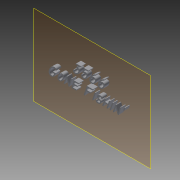
# Autodesk Inventor part: RaisedLetters3566GF
Saved by Autodesk Inventor 2015 (Build 190159000, 159)
## iProperties
Created: 2016-02-29
Part Number: RaisedLetters3566GF
Material: Generic
Document SubType Name: Modeling
Designer: robotics
Density: 1 g/cm^3
Appearance: Default
Author: robotics
Autodesk Inventor part; units mm, degrees
ref_plane "YZ Plane" through (0, 0, 0) normal (1, 0, 0) x (0, 1, 0)
ref_plane "XZ Plane" through (0, 0, 0) normal (0, 1, 0) x (-1, 0, 0)
ref_plane "XY Plane" through (0, 0, 0) normal (0, 0, 1) x (1, 0, 0)
sketch "Sketch1" plane through (0, 0, 0) normal (0, 0, 1) x (1, 0, 0)
  line L0 (0, 0) -> (127, 0)
  line L1 (127, 0) -> (127, 76.2)
  line L2 (127, 76.2) -> (0, 76.2)
  line L3 (0, 76.2) -> (0, 0)
  line L4 (3.7507, 56.7748) -> (124.5302, 56.7748) construction
  line L5 (124.5302, 56.7748) -> (124.5302, -11.4457) construction
  line L6 (124.5302, -11.4457) -> (3.7507, -11.4457) construction
  line L7 (3.7507, -11.4457) -> (3.7507, 56.7748) construction
  spline S0 degree 2 poles (52.7475, 48.5617) (52.0257, 46.4353) (50.3285, 45.138) knots 0 0 0 1 1 1
  spline S1 degree 2 poles (50.3285, 45.138) (48.7873, 43.9772) (47.1681, 43.9772) knots 0 0 0 1 1 1
  spline S2 degree 2 poles (47.1681, 43.9772) (45.9098, 43.9772) (45.1685, 44.7186) knots 0 0 0 1 1 1
  spline S3 degree 2 poles (45.1685, 44.7186) (44.3491, 45.5282) (44.3882, 46.9913) knots 0 0 0 1 1 1
  spline S4 degree 2 poles (44.3882, 46.9913) (44.3979, 47.1181) (44.4369, 47.2449) knots 0 0 0 1 1 1
  spline S5 degree 2 poles (44.4369, 47.2449) (44.554, 47.5765) (45.149, 47.9862) (45.4416, 47.9862) knots 0 0 0 1 2 2 2
  spline S6 degree 2 poles (45.4416, 47.9862) (45.9586, 47.9862) (45.9488, 47.4692) knots 0 0 0 1 1 1
  spline S7 degree 2 poles (45.9488, 47.4692) (45.9196, 46.5621) (46.4268, 46.0451) knots 0 0 0 1 1 1
  spline S8 degree 2 poles (46.4268, 46.0451) (46.9048, 45.5867) (47.6753, 45.5867) knots 0 0 0 1 1 1
  spline S9 degree 2 poles (47.6753, 45.5867) (48.7093, 45.5867) (49.714, 46.3573) knots 0 0 0 1 1 1
  spline S10 degree 2 poles (49.714, 46.3573) (50.8064, 47.1961) (51.2746, 48.5617) knots 0 0 0 1 1 1
  spline S11 degree 2 poles (51.2746, 48.5617) (51.7721, 50.0151) (51.1771, 50.7759) knots 0 0 0 1 1 1
  spline S12 degree 2 poles (51.1771, 50.7759) (50.7284, 51.3027) (49.7335, 51.4685) knots 0 0 0 1 1 1
  spline S13 degree 2 poles (49.7335, 51.4685) (49.1872, 51.5075) (48.6313, 51.5465) knots 0 0 0 1 1 1
  spline S14 degree 2 poles (48.6313, 51.5465) (48.3289, 51.566) (48.046, 51.9562) (48.1143, 52.1513) knots 0 0 0 1 2 2 2
  spline S15 degree 2 poles (48.1143, 52.1513) (48.2411, 52.5219) (48.6703, 52.8536) knots 0 0 0 1 1 1
  line L8 (48.6703, 52.8536) -> (51.577, 55.1068)
  line L9 (51.577, 55.1068) -> (48.3874, 55.1068)
  spline S16 degree 2 poles (48.3874, 55.1068) (47.6461, 55.1068) (47.8997, 55.8676) knots 0 0 0 1 1 1
  spline S17 degree 2 poles (47.8997, 55.8676) (48.163, 56.6382) (48.9044, 56.6382) knots 0 0 0 1 1 1
  line L10 (48.9044, 56.6382) -> (54.5033, 56.6577)
  spline S18 degree 2 poles (54.5033, 56.6577) (55.0203, 56.6577) (54.8935, 56.2773) knots 0 0 0 1 1 1
  spline S19 degree 2 poles (54.8935, 56.2773) (54.7959, 55.9944) (53.8888, 55.3019) knots 0 0 0 1 1 1
  line L11 (53.8888, 55.3019) -> (50.904, 52.9706)
  spline S20 degree 2 poles (50.904, 52.9706) (54.0156, 52.3073) (52.7475, 48.5617) knots 0 0 0 1 1 1
  spline S21 degree 2 poles (63.1065, 48.4056) (62.4725, 46.5426) (61.2044, 45.3623) knots 0 0 0 1 1 1
  spline S22 degree 2 poles (61.2044, 45.3623) (59.8096, 44.0845) (57.9758, 43.9577) knots 0 0 0 1 1 1
  spline S23 degree 2 poles (57.9758, 43.9577) (56.5322, 43.8504) (55.7421, 44.7673) knots 0 0 0 1 1 1
  spline S24 degree 2 poles (55.7421, 44.7673) (55.0105, 45.6062) (55.0008, 47.0401) knots 0 0 0 1 1 1
  spline S25 degree 2 poles (55.0008, 47.0401) (54.991, 47.1864) (55.0398, 47.3327) knots 0 0 0 1 1 1
  spline S26 degree 2 poles (55.0398, 47.3327) (55.1471, 47.6546) (55.7713, 48.074) (56.0835, 48.074) knots 0 0 0 1 2 2 2
  spline S27 degree 2 poles (56.0835, 48.074) (56.5712, 48.074) (56.5809, 47.5765) knots 0 0 0 1 1 1
  spline S28 degree 2 poles (56.5809, 47.5765) (56.6395, 45.4013) (58.4147, 45.5086) knots 0 0 0 1 1 1
  spline S29 degree 2 poles (58.4147, 45.5086) (59.5462, 45.5867) (60.4241, 46.4353) knots 0 0 0 1 1 1
  spline S30 degree 2 poles (60.4241, 46.4353) (61.224, 47.2059) (61.6336, 48.4056) knots 0 0 0 1 1 1
  spline S31 degree 2 poles (61.6336, 48.4056) (62.0238, 49.5762) (61.1264, 51.2734) (60.151, 51.2734) knots 0 0 0 1 2 2 2
  spline S32 degree 2 poles (60.151, 51.2734) (58.8049, 51.2734) (57.7222, 50.5906) knots 0 0 0 1 1 1
  spline S33 degree 2 poles (57.7222, 50.5906) (57.176, 50.2394) (56.9028, 50.2394) knots 0 0 0 1 1 1
  spline S34 degree 2 poles (56.9028, 50.2394) (56.2883, 50.2394) (56.5224, 50.9222) knots 0 0 0 1 1 1
  line L12 (56.5224, 50.9222) -> (58.4733, 56.648)
  line L13 (58.4733, 56.648) -> (64.2283, 56.648)
  spline S35 degree 2 poles (64.2283, 56.648) (64.9793, 56.648) (64.7257, 55.8871) knots 0 0 0 1 1 1
  spline S36 degree 2 poles (64.7257, 55.8871) (64.4624, 55.1166) (63.7015, 55.1166) knots 0 0 0 1 1 1
  line L14 (63.7015, 55.1166) -> (59.4194, 55.1166)
  line L15 (59.4194, 55.1166) -> (58.522, 52.4537)
  spline S37 degree 2 poles (58.522, 52.4537) (59.4877, 52.8243) (60.6777, 52.8243) knots 0 0 0 1 1 1
  spline S38 degree 2 poles (60.6777, 52.8243) (62.2091, 52.8243) (63.7113, 50.2004) (63.1065, 48.4056) knots 0 0 0 1 2 2 2
  spline S39 degree 2 poles (74.4604, 48.5715) (73.7679, 46.5231) (70.6758, 43.8992) (68.9103, 43.8992) knots 0 0 0 1 2 2 2
  spline S40 degree 2 poles (68.9103, 43.8992) (66.6961, 43.8992) (66.0425, 45.4696) knots 0 0 0 1 1 1
  spline S41 degree 2 poles (66.0425, 45.4696) (65.4573, 46.8352) (66.1889, 49.0007) knots 0 0 0 1 1 1
  spline S42 degree 2 poles (66.1889, 49.0007) (66.5693, 50.1224) (67.2618, 51.2344) knots 0 0 0 1 1 1
  spline S43 degree 2 poles (67.2618, 51.2344) (68.3543, 52.9706) (69.7101, 54.1899) knots 0 0 0 1 1 1
  spline S44 degree 2 poles (69.7101, 54.1899) (71.1928, 55.5165) (73.485, 56.6675) knots 0 0 0 1 1 1
  spline S45 degree 2 poles (73.485, 56.6675) (73.7094, 56.7748) (73.8947, 56.7748) knots 0 0 0 1 1 1
  spline S46 degree 2 poles (73.8947, 56.7748) (74.2068, 56.7748) (74.4604, 56.2773) (74.3531, 55.9652) knots 0 0 0 1 2 2 2
  spline S47 degree 2 poles (74.3531, 55.9652) (74.2068, 55.536) (73.7679, 55.3116) knots 0 0 0 1 1 1
  spline S48 degree 2 poles (73.7679, 55.3116) (72.4511, 54.6484) (71.4952, 53.907) knots 0 0 0 1 1 1
  spline S49 degree 2 poles (71.4952, 53.907) (70.6563, 53.2828) (69.515, 52.1415) knots 0 0 0 1 1 1
  spline S50 degree 2 poles (69.515, 52.1415) (70.5783, 52.6878) (71.7975, 52.6878) knots 0 0 0 1 1 1
  spline S51 degree 2 poles (71.7975, 52.6878) (73.7191, 52.6878) (75.1237, 50.5321) (74.4604, 48.5715) knots 0 0 0 1 2 2 2
  spline S52 degree 2 poles (72.968, 48.5715) (73.3289, 49.6249) (72.3243, 51.1368) (71.2708, 51.1368) knots 0 0 0 1 2 2 2
  spline S53 degree 2 poles (71.2708, 51.1368) (70.1491, 51.1368) (67.9934, 49.4786) (67.5935, 48.2984) knots 0 0 0 1 2 2 2
  spline S54 degree 2 poles (67.5935, 48.2984) (67.1838, 47.1083) (68.2665, 45.4501) (69.437, 45.4501) knots 0 0 0 1 2 2 2
  spline S55 degree 2 poles (69.437, 45.4501) (70.5197, 45.4501) (71.5732, 46.4255) knots 0 0 0 1 1 1
  spline S56 degree 2 poles (71.5732, 46.4255) (72.5486, 47.3327) (72.968, 48.5715) knots 0 0 0 1 1 1
  spline S57 degree 2 poles (85.5705, 48.5715) (84.8779, 46.5231) (81.7859, 43.8992) (80.0203, 43.8992) knots 0 0 0 1 2 2 2
  spline S58 degree 2 poles (80.0203, 43.8992) (77.8061, 43.8992) (77.1526, 45.4696) knots 0 0 0 1 1 1
  spline S59 degree 2 poles (77.1526, 45.4696) (76.5673, 46.8352) (77.2989, 49.0007) knots 0 0 0 1 1 1
  spline S60 degree 2 poles (77.2989, 49.0007) (77.6793, 50.1224) (78.3719, 51.2344) knots 0 0 0 1 1 1
  spline S61 degree 2 poles (78.3719, 51.2344) (79.4644, 52.9706) (80.8202, 54.1899) knots 0 0 0 1 1 1
  spline S62 degree 2 poles (80.8202, 54.1899) (82.3028, 55.5165) (84.5951, 56.6675) knots 0 0 0 1 1 1
  spline S63 degree 2 poles (84.5951, 56.6675) (84.8194, 56.7748) (85.0048, 56.7748) knots 0 0 0 1 1 1
  spline S64 degree 2 poles (85.0048, 56.7748) (85.3169, 56.7748) (85.5705, 56.2773) (85.4632, 55.9652) knots 0 0 0 1 2 2 2
  spline S65 degree 2 poles (85.4632, 55.9652) (85.3169, 55.536) (84.8779, 55.3116) knots 0 0 0 1 1 1
  spline S66 degree 2 poles (84.8779, 55.3116) (83.5611, 54.6484) (82.6052, 53.907) knots 0 0 0 1 1 1
  spline S67 degree 2 poles (82.6052, 53.907) (81.7664, 53.2828) (80.6251, 52.1415) knots 0 0 0 1 1 1
  spline S68 degree 2 poles (80.6251, 52.1415) (81.6883, 52.6878) (82.9076, 52.6878) knots 0 0 0 1 1 1
  spline S69 degree 2 poles (82.9076, 52.6878) (84.8292, 52.6878) (86.2338, 50.5321) (85.5705, 48.5715) knots 0 0 0 1 2 2 2
  spline S70 degree 2 poles (84.0781, 48.5715) (84.439, 49.6249) (83.4343, 51.1368) (82.3809, 51.1368) knots 0 0 0 1 2 2 2
  spline S71 degree 2 poles (82.3809, 51.1368) (81.2591, 51.1368) (79.1034, 49.4786) (78.7035, 48.2984) knots 0 0 0 1 2 2 2
  spline S72 degree 2 poles (78.7035, 48.2984) (78.2938, 47.1083) (79.3766, 45.4501) (80.5471, 45.4501) knots 0 0 0 1 2 2 2
  spline S73 degree 2 poles (80.5471, 45.4501) (81.6298, 45.4501) (82.6832, 46.4255) knots 0 0 0 1 1 1
  spline S74 degree 2 poles (82.6832, 46.4255) (83.6587, 47.3327) (84.0781, 48.5715) knots 0 0 0 1 1 1
  spline S75 degree 2 poles (20.9439, 30.1166) (20.0758, 27.5708) (18.2712, 26.332) knots 0 0 0 1 1 1
  spline S76 degree 2 poles (18.2712, 26.332) (16.9934, 25.4638) (15.7059, 25.4638) knots 0 0 0 1 1 1
  spline S77 degree 2 poles (15.7059, 25.4638) (13.4819, 25.4638) (12.7211, 27.5122) knots 0 0 0 1 1 1
  spline S78 degree 2 poles (12.7211, 27.5122) (12.009, 29.3753) (12.8284, 31.8041) knots 0 0 0 1 1 1
  spline S79 degree 2 poles (12.8284, 31.8041) (13.8428, 34.7694) (15.8619, 36.5837) knots 0 0 0 1 1 1
  spline S80 degree 2 poles (15.8619, 36.5837) (17.7835, 38.3394) (19.8709, 38.3394) knots 0 0 0 1 1 1
  spline S81 degree 2 poles (19.8709, 38.3394) (21.3341, 38.3394) (22.0071, 37.7347) knots 0 0 0 1 1 1
  spline S82 degree 2 poles (22.0071, 37.7347) (22.407, 37.3835) (22.6996, 36.4569) knots 0 0 0 1 1 1
  spline S83 degree 2 poles (22.6996, 36.4569) (22.7874, 36.213) (22.6996, 35.9594) knots 0 0 0 1 1 1
  spline S84 degree 2 poles (22.6996, 35.9594) (22.6021, 35.657) (21.9973, 35.2376) (21.695, 35.2376) knots 0 0 0 1 2 2 2
  spline S85 degree 2 poles (21.695, 35.2376) (21.3145, 35.2376) (21.1682, 35.5887) knots 0 0 0 1 1 1
  spline S86 degree 2 poles (21.1682, 35.5887) (20.9244, 36.2325) (20.6805, 36.4373) knots 0 0 0 1 1 1
  spline S87 degree 2 poles (20.6805, 36.4373) (20.2904, 36.7885) (19.3442, 36.7885) knots 0 0 0 1 1 1
  spline S88 degree 2 poles (19.3442, 36.7885) (17.8518, 36.7885) (15.1011, 34.0378) (14.3403, 31.8041) knots 0 0 0 1 2 2 2
  spline S89 degree 2 poles (14.3403, 31.8041) (13.7258, 29.9898) (14.1549, 28.5852) knots 0 0 0 1 1 1
  spline S90 degree 2 poles (14.1549, 28.5852) (14.6427, 27.0148) (16.2228, 27.0148) knots 0 0 0 1 1 1
  spline S91 degree 2 poles (16.2228, 27.0148) (17.6274, 27.0148) (18.5346, 28.3804) knots 0 0 0 1 1 1
  spline S92 degree 2 poles (18.5346, 28.3804) (19.0223, 29.0827) (19.5198, 30.5653) knots 0 0 0 1 1 1
  line L16 (19.5198, 30.5653) -> (17.842, 30.5653)
  spline S93 degree 2 poles (17.842, 30.5653) (17.0617, 30.5653) (17.3251, 31.3456) knots 0 0 0 1 1 1
  spline S94 degree 2 poles (17.3251, 31.3456) (17.5884, 32.1162) (18.3688, 32.1162) knots 0 0 0 1 1 1
  line L17 (18.3688, 32.1162) -> (21.6169, 32.1162)
  line L18 (21.6169, 32.1162) -> (20.9439, 30.1166)
  spline S95 degree 2 poles (32.0344, 30.7506) (31.3419, 28.7218) (29.8007, 27.1806) knots 0 0 0 1 1 1
  spline S96 degree 2 poles (29.8007, 27.1806) (28.1327, 25.5224) (26.416, 25.5224) knots 0 0 0 1 1 1
  spline S97 degree 2 poles (26.416, 25.5224) (24.6993, 25.5224) (24.1628, 27.2001) knots 0 0 0 1 1 1
  spline S98 degree 2 poles (24.1628, 27.2001) (23.6751, 28.7315) (24.3579, 30.7506) knots 0 0 0 1 1 1
  spline S99 degree 2 poles (24.3579, 30.7506) (25.0407, 32.76) (26.6013, 34.2719) knots 0 0 0 1 1 1
  spline S100 degree 2 poles (26.6013, 34.2719) (28.2888, 35.9204) (29.947, 35.9204) knots 0 0 0 1 1 1
  spline S101 degree 2 poles (29.947, 35.9204) (31.7223, 35.9204) (32.249, 34.2719) knots 0 0 0 1 1 1
  spline S102 degree 2 poles (32.249, 34.2719) (32.727, 32.799) (32.0344, 30.7506) knots 0 0 0 1 1 1
  spline S103 degree 2 poles (30.5615, 30.7506) (31.059, 32.2138) (30.8542, 33.2087) knots 0 0 0 1 1 1
  spline S104 degree 2 poles (30.8542, 33.2087) (30.6201, 34.4085) (29.4398, 34.4085) knots 0 0 0 1 1 1
  spline S105 degree 2 poles (29.4398, 34.4085) (28.3083, 34.4085) (27.2354, 33.2087) knots 0 0 0 1 1 1
  spline S106 degree 2 poles (27.2354, 33.2087) (26.3087, 32.1748) (25.8308, 30.7506) knots 0 0 0 1 1 1
  spline S107 degree 2 poles (25.8308, 30.7506) (25.343, 29.3265) (25.5576, 28.2731) knots 0 0 0 1 1 1
  spline S108 degree 2 poles (25.5576, 28.2731) (25.7917, 27.0538) (26.933, 27.0538) knots 0 0 0 1 1 1
  spline S109 degree 2 poles (26.933, 27.0538) (28.084, 27.0538) (29.1472, 28.2731) knots 0 0 0 1 1 1
  spline S110 degree 2 poles (29.1472, 28.2731) (30.0738, 29.3265) (30.5615, 30.7506) knots 0 0 0 1 1 1
  spline S111 degree 2 poles (39.8086, 26.3515) (39.5354, 25.5614) (38.9112, 25.5614) knots 0 0 0 1 1 1
  spline S112 degree 2 poles (38.9112, 25.5614) (38.4625, 25.5614) (38.2869, 26.0784) knots 0 0 0 1 1 1
  line L19 (38.2869, 26.0784) -> (35.9654, 32.8966)
  line L20 (35.9654, 32.8966) -> (33.7414, 26.332)
  spline S113 degree 2 poles (33.7414, 26.332) (33.4781, 25.5614) (32.7367, 25.5614) knots 0 0 0 1 1 1
  spline S114 degree 2 poles (32.7367, 25.5614) (32.0052, 25.5614) (32.2685, 26.332) knots 0 0 0 1 1 1
  line L21 (32.2685, 26.332) -> (35.2923, 35.2376)
  spline S115 degree 2 poles (35.2923, 35.2376) (35.546, 35.9887) (36.2483, 35.9887) knots 0 0 0 1 1 1
  spline S116 degree 2 poles (36.2483, 35.9887) (36.697, 35.9887) (36.853, 35.5302) knots 0 0 0 1 1 1
  line L22 (36.853, 35.5302) -> (39.155, 28.7705)
  line L23 (39.155, 28.7705) -> (41.3205, 35.1595)
  spline S117 degree 2 poles (41.3205, 35.1595) (41.5936, 35.9399) (42.3251, 35.9399) knots 0 0 0 1 1 1
  spline S118 degree 2 poles (42.3251, 35.9399) (43.0665, 35.9399) (42.7933, 35.1595) knots 0 0 0 1 1 1
  line L24 (42.7933, 35.1595) -> (39.8086, 26.3515)
  line L25 (48.0801, 25.7077) -> (42.0423, 25.7077)
  line L26 (42.0423, 25.7077) -> (45.5245, 35.9399)
  line L27 (45.5245, 35.9399) -> (51.5624, 35.9399)
  spline S119 degree 2 poles (51.5624, 35.9399) (52.3135, 35.9399) (52.0599, 35.1888) knots 0 0 0 1 1 1
  spline S120 degree 2 poles (52.0599, 35.1888) (51.7965, 34.428) (51.0454, 34.428) knots 0 0 0 1 1 1
  line L28 (51.0454, 34.428) -> (46.4707, 34.428)
  line L29 (46.4707, 34.428) -> (45.6806, 32.1162)
  line L30 (45.6806, 32.1162) -> (49.9822, 32.1162)
  spline S121 degree 2 poles (49.9822, 32.1162) (50.7235, 32.1162) (50.4602, 31.3554) knots 0 0 0 1 1 1
  spline S122 degree 2 poles (50.4602, 31.3554) (50.1968, 30.5848) (49.4652, 30.5848) knots 0 0 0 1 1 1
  line L31 (49.4652, 30.5848) -> (45.1636, 30.5848)
  line L32 (45.1636, 30.5848) -> (44.0224, 27.2391)
  line L33 (44.0224, 27.2391) -> (48.5971, 27.2391)
  spline S123 degree 2 poles (48.5971, 27.2391) (49.3579, 27.2391) (49.1043, 26.4783) knots 0 0 0 1 1 1
  spline S124 degree 2 poles (49.1043, 26.4783) (48.841, 25.7077) (48.0801, 25.7077) knots 0 0 0 1 1 1
  line L34 (69.5687, 36.6617) -> (63.5113, 36.6617)
  line L35 (63.5113, 36.6617) -> (62.3798, 33.355)
  line L36 (62.3798, 33.355) -> (67.0228, 33.355)
  spline S125 degree 2 poles (67.0228, 33.355) (67.7837, 33.355) (67.5203, 32.5844) knots 0 0 0 1 1 1
  spline S126 degree 2 poles (67.5203, 32.5844) (67.2472, 31.8041) (66.4961, 31.8041) knots 0 0 0 1 1 1
  line L37 (66.4961, 31.8041) -> (61.8531, 31.8041)
  line L38 (61.8531, 31.8041) -> (60.0193, 26.3905)
  spline S127 degree 2 poles (60.0193, 26.3905) (59.7462, 25.6004) (59.0146, 25.6004) knots 0 0 0 1 1 1
  spline S128 degree 2 poles (59.0146, 25.6004) (58.2538, 25.6004) (58.5269, 26.3905) knots 0 0 0 1 1 1
  line L39 (58.5269, 26.3905) -> (62.5457, 38.2126)
  line L40 (62.5457, 38.2126) -> (70.0954, 38.2126)
  spline S129 degree 2 poles (70.0954, 38.2126) (70.8562, 38.2126) (70.5929, 37.442) knots 0 0 0 1 1 1
  spline S130 degree 2 poles (70.5929, 37.442) (70.3198, 36.6617) (69.5687, 36.6617) knots 0 0 0 1 1 1
  spline S131 degree 2 poles (71.0904, 26.3612) (70.827, 25.5809) (70.0662, 25.5809) knots 0 0 0 1 1 1
  spline S132 degree 2 poles (70.0662, 25.5809) (69.3151, 25.5809) (69.5784, 26.3612) knots 0 0 0 1 1 1
  line L41 (69.5784, 26.3612) -> (72.573, 35.1791)
  spline S133 degree 2 poles (72.573, 35.1791) (72.8364, 35.9594) (73.5972, 35.9594) knots 0 0 0 1 1 1
  spline S134 degree 2 poles (73.5972, 35.9594) (74.3483, 35.9594) (74.0849, 35.1791) knots 0 0 0 1 1 1
  line L42 (74.0849, 35.1791) -> (71.0904, 26.3612)
  spline S135 degree 2 poles (81.4103, 28.5169) (80.3861, 25.5029) (76.6503, 25.5029) knots 0 0 0 1 1 1
  spline S136 degree 2 poles (76.6503, 25.5029) (74.5433, 25.5029) (74.1044, 27.7171) knots 0 0 0 1 1 1
  spline S137 degree 2 poles (74.1044, 27.7171) (74.0654, 27.8829) (74.1239, 28.0682) knots 0 0 0 1 1 1
  spline S138 degree 2 poles (74.1239, 28.0682) (74.2507, 28.4194) (74.9628, 28.9559) (75.2749, 28.9559) knots 0 0 0 1 2 2 2
  spline S139 degree 2 poles (75.2749, 28.9559) (75.6261, 28.9559) (75.6651, 28.5657) knots 0 0 0 1 1 1
  spline S140 degree 2 poles (75.6651, 28.5657) (75.7724, 27.0343) (77.177, 27.0343) knots 0 0 0 1 1 1
  spline S141 degree 2 poles (77.177, 27.0343) (79.3912, 27.0343) (79.8887, 28.4974) knots 0 0 0 1 1 1
  spline S142 degree 2 poles (79.8887, 28.4974) (80.113, 29.1607) (78.9035, 29.7655) knots 0 0 0 1 1 1
  spline S143 degree 2 poles (78.9035, 29.7655) (76.9819, 30.7116) (76.66, 30.975) knots 0 0 0 1 1 1
  spline S144 degree 2 poles (76.66, 30.975) (75.5578, 31.8919) (76.0553, 33.3745) knots 0 0 0 1 1 1
  spline S145 degree 2 poles (76.0553, 33.3745) (76.9429, 35.9984) (80.152, 36.1447) knots 0 0 0 1 1 1
  spline S146 degree 2 poles (80.152, 36.1447) (81.3713, 36.2032) (82.8735, 35.0522) (82.8539, 33.9305) knots 0 0 0 1 2 2 2
  spline S147 degree 2 poles (82.8539, 33.9305) (82.8539, 33.794) (82.8052, 33.6671) knots 0 0 0 1 1 1
  spline S148 degree 2 poles (82.8052, 33.6671) (82.7076, 33.3745) (82.1321, 32.9844) (81.8298, 32.9844) knots 0 0 0 1 2 2 2
  spline S149 degree 2 poles (81.8298, 32.9844) (81.2933, 32.9844) (81.3128, 34.0573) (80.4154, 34.6718) (79.7131, 34.6328) knots 0 0 0 1 2 3 3 3
  spline S150 degree 2 poles (79.7131, 34.6328) (77.9671, 34.5548) (77.5769, 33.4135) knots 0 0 0 1 1 1
  spline S151 degree 2 poles (77.5769, 33.4135) (77.2648, 32.4869) (78.4743, 31.8626) knots 0 0 0 1 1 1
  spline S152 degree 2 poles (78.4743, 31.8626) (79.6058, 31.3066) (80.7373, 30.7311) knots 0 0 0 1 1 1
  spline S153 degree 2 poles (80.7373, 30.7311) (81.8883, 29.9215) (81.4103, 28.5169) knots 0 0 0 1 1 1
  spline S154 degree 2 poles (89.994, 26.3612) (89.7307, 25.5809) (88.9894, 25.5809) knots 0 0 0 1 1 1
  spline S155 degree 2 poles (88.9894, 25.5809) (88.2383, 25.5809) (88.5016, 26.3515) knots 0 0 0 1 1 1
  line L43 (88.5016, 26.3515) -> (89.838, 30.3019)
  line L44 (89.838, 30.3019) -> (85.7314, 30.3019)
  line L45 (85.7314, 30.3019) -> (84.3951, 26.3515)
  spline S156 degree 2 poles (84.3951, 26.3515) (84.1317, 25.5809) (83.3709, 25.5809) knots 0 0 0 1 1 1
  spline S157 degree 2 poles (83.3709, 25.5809) (82.6198, 25.5809) (82.8832, 26.3612) knots 0 0 0 1 1 1
  line L46 (82.8832, 26.3612) -> (85.8778, 35.1791)
  spline S158 degree 2 poles (85.8778, 35.1791) (86.1411, 35.9594) (86.9019, 35.9594) knots 0 0 0 1 1 1
  spline S159 degree 2 poles (86.9019, 35.9594) (87.653, 35.9594) (87.3897, 35.1791) knots 0 0 0 1 1 1
  line L47 (87.3897, 35.1791) -> (86.2484, 31.8334)
  line L48 (86.2484, 31.8334) -> (90.3549, 31.8334)
  line L49 (90.3549, 31.8334) -> (91.4962, 35.1791)
  spline S160 degree 2 poles (91.4962, 35.1791) (91.7596, 35.9594) (92.5204, 35.9594) knots 0 0 0 1 1 1
  spline S161 degree 2 poles (92.5204, 35.9594) (93.2519, 35.9594) (92.9886, 35.1791) knots 0 0 0 1 1 1
  line L50 (92.9886, 35.1791) -> (89.994, 26.3612)
  spline S162 degree 2 poles (94.0908, 26.3612) (93.8274, 25.5809) (93.0666, 25.5809) knots 0 0 0 1 1 1
  spline S163 degree 2 poles (93.0666, 25.5809) (92.3155, 25.5809) (92.5789, 26.3612) knots 0 0 0 1 1 1
  line L51 (92.5789, 26.3612) -> (95.5735, 35.1791)
  spline S164 degree 2 poles (95.5735, 35.1791) (95.8368, 35.9594) (96.5976, 35.9594) knots 0 0 0 1 1 1
  spline S165 degree 2 poles (96.5976, 35.9594) (97.3487, 35.9594) (97.0854, 35.1791) knots 0 0 0 1 1 1
  line L52 (97.0854, 35.1791) -> (94.0908, 26.3612)
  spline S166 degree 2 poles (104.3327, 26.3515) (104.0596, 25.5614) (103.4354, 25.5614) knots 0 0 0 1 1 1
  spline S167 degree 2 poles (103.4354, 25.5614) (102.9867, 25.5614) (102.8111, 26.0784) knots 0 0 0 1 1 1
  line L53 (102.8111, 26.0784) -> (100.4896, 32.8966)
  line L54 (100.4896, 32.8966) -> (98.2656, 26.332)
  spline S168 degree 2 poles (98.2656, 26.332) (98.0023, 25.5614) (97.2609, 25.5614) knots 0 0 0 1 1 1
  spline S169 degree 2 poles (97.2609, 25.5614) (96.5294, 25.5614) (96.7927, 26.332) knots 0 0 0 1 1 1
  line L55 (96.7927, 26.332) -> (99.8165, 35.2376)
  spline S170 degree 2 poles (99.8165, 35.2376) (100.0702, 35.9887) (100.7725, 35.9887) knots 0 0 0 1 1 1
  spline S171 degree 2 poles (100.7725, 35.9887) (101.2211, 35.9887) (101.3772, 35.5302) knots 0 0 0 1 1 1
  line L56 (101.3772, 35.5302) -> (103.6792, 28.7705)
  line L57 (103.6792, 28.7705) -> (105.8447, 35.1595)
  spline S172 degree 2 poles (105.8447, 35.1595) (106.1178, 35.9399) (106.8493, 35.9399) knots 0 0 0 1 1 1
  spline S173 degree 2 poles (106.8493, 35.9399) (107.5907, 35.9399) (107.3175, 35.1595) knots 0 0 0 1 1 1
  line L58 (107.3175, 35.1595) -> (104.3327, 26.3515)
  spline S174 degree 2 poles (111.8337, 34.7401) (111.5996, 34.0573) (110.8388, 34.0573) knots 0 0 0 1 1 1
  spline S175 degree 2 poles (110.8388, 34.0573) (110.0877, 34.0573) (110.3218, 34.7401) knots 0 0 0 1 1 1
  line L59 (110.3218, 34.7401) -> (111.268, 37.5396)
  spline S176 degree 2 poles (111.268, 37.5396) (111.5021, 38.2224) (112.2629, 38.2224) knots 0 0 0 1 1 1
  spline S177 degree 2 poles (112.2629, 38.2224) (113.014, 38.2224) (112.7799, 37.5396) knots 0 0 0 1 1 1
  line L60 (112.7799, 37.5396) -> (111.8337, 34.7401)
  dimension "d0" = 127
  dimension "d1" = 76.2
  constraints: 8 end point, 2 parallel, 1 horizontal, 1 perpendicular, 2 other
  measures "d0" distance of L1.end L2.end
  measures "d1" distance of L2.end L0.start
ref_plane "Work Plane1" through (127, 76.2, 0) normal (0, 0, 1) x (-1, 0, 0)
extrude "Extrusion1" add sketch "Sketch1" along normal blind 6.35 contours S0 S1 S2 S3 S4 S5 S6 S7 S8 S9 S10 S11 S12 S13 S14 S15 L8 L9 S16 S17 L10 S18 S19 L11 S20 | S21 S22 S23 S24 S25 S26 S27 S28 S29 S30 S31 S32 S33 S34 L12 L13 S35 S36 L14 L15 S37 S38 | S39 S40 S41 S42 S43 S44 S45 S46 S47 S48 S49 S50 S51 | S57 S58 S59 S60 S61 S62 S63 S64 S65 S66 S67 S68 S69 | S75 S76 S77 S78 S79 S80 S81 S82 S83 S84 S85 S86 S87 S88 S89 S90 S91 S92 L16 S93 S94 L17 L18 | S95 S96 S97 S98 S99 S100 S101 S102 | S111 S112 L19 L20 S113 S114 L21 S115 S116 L22 L23 S117 S118 L24 | L25 L26 L27 S119 S120 L28 L29 L30 S121 S122 L31 L32 L33 S123 S124 | L34 L35 L36 S125 S126 L37 L38 S127 S128 L39 L40 S129 S130 | S131 S132 L41 S133 S134 L42 | S135 S136 S137 S138 S139 S140 S141 S142 S143 S144 S145 S146 S147 S148 S149 S150 S151 S152 S153 | S154 S155 L43 L44 L45 S156 S157 L46 S158 S159 L47 L48 L49 S160 S161 L50 | S162 S163 L51 S164 S165 L52 | S166 S167 L53 L54 S168 S169 L55 S170 S171 L56 L57 S172 S173 L58 | S174 S175 L59 S176 S177 L60
body "Solid1"
